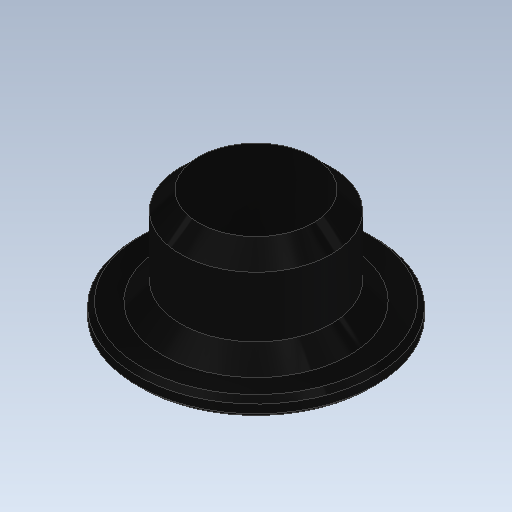
# Autodesk Inventor part: Base Plate
Saved by Autodesk Inventor 2020 (Build 240168000, 168)
## iProperties
Created: 2012-10-13
Part Number: Base Plate
Material: Steel, Mild
Document SubType Name: Modeling
Designer: Lance
Mass: 81.4592 g
Surface Area: 41.1888 cm^2
Volume: 10.377 cm^3
Density: 7.85 g/cm^3
Appearance: Glossy - Black
Author: Lance
Autodesk Inventor part; units mm, degrees
ref_plane "YZ Plane" through (0, 0, 0) normal (1, 0, 0) x (0, 1, 0)
ref_plane "XZ Plane" through (0, 0, 0) normal (0, 1, 0) x (-1, 0, 0)
ref_plane "XY Plane" through (0, 0, 0) normal (0, 0, 1) x (1, 0, 0)
sketch "Sketch1" plane through (0, 0, 0) normal (0, 0, 1) x (1, 0, 0)
  line L0 (0, -5.3) -> (0, 21.3) projected
  line L1 (0, 17.5) -> (-12.5, 17.5)
  line L2 (-12.5, 17.5) -> (-12.5, 1.5)
  line L3 (-12.5, 1.5) -> (-19.75, 1.5)
  line L4 (-19.75, 1.5) -> (-19.75, -1.5)
  line L5 (-19.75, -1.5) -> (-13.5, -1.5)
  line L6 (-13.5, -1.5) -> (-13.5, -1)
  line L7 (-13.5, -1) -> (0, -1)
  point P0 (0, 0)
  point P1 (-19.75, 0)
  dimension "d0" = 39.5
  dimension "d1" = 25
  dimension "d2" = 3
  dimension "d3" = 16
  dimension "d4" = 27
  dimension "d5" = 0.5
  constraints: 14 end point, 5 perpendicular, 2 parallel, 2 point on line, 1 horizontal alignment, 1 midpoint
  measures "d0" diameter of L4 L0
  measures "d1" diameter of L2 L0
  measures "d2" distance between parallel lines of L5 L3
  measures "d3" distance between parallel lines of L3 L1
  measures "d4" diameter of L6 L0
  measures "d5" distance between parallel lines of L5 L7
revolve "Revolution1" add sketch "Sketch1" angle 360 about axis through (0, -10, 0) along (0, 1, 0)
sketch "Sketch2" plane through (0, -1.5, 0) normal (0, -1, 0) x (1, 0, 0)
  point P0 (0, 0)
  point P1 (0, 0)
  constraints: 1 coincident
hole "Hole1" at (0, -1.5, 0) direction (0, 1, 0) diameter 8.376 depth 15 tip angle 118 thread size "M10x1.5" class "6H" standard "ISO Metric profile"
chamfer "Chamfer1" distance 3 angle 45 1 edges at (12.5, 1.5, 0)
chamfer "Chamfer2" distance 0.8 angle 45 2 edges at (19.75, 1.5, 0) (19.75, -1.5, 0)
chamfer "Chamfer3" distance 3 angle 45 1 edges at (12.5, 17.5, 0)
body "Solid1"
